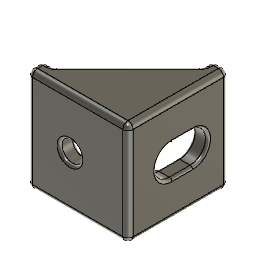
1) Custom PLA Corner Bracket (Autodesk Fusion 360 design; units mm, degrees)
Autodesk Fusion 360 part; units mm, degrees
ref_plane "WorkPlane1" through (0, 0, 0) normal (0, 0, 1) x (1, 0, 0)
sketch "Sketch1" plane through (0, 0, 0) normal (0, 0, 1) x (1, 0, 0)
  line L0 (0, 0) -> (19.5, 0)
  line L1 (19.5, 0) -> (19.5, 19.5)
  line L2 (19.5, 19.5) -> (0, 19.5)
  line L3 (0, 19.5) -> (0, 0)
  line L4 (0, 3) -> (2, 3)
  line L5 (2, 3) -> (16.5, 17.5)
  line L6 (16.5, 17.5) -> (16.5, 19.5)
  dimension "d2" = 19.5
  dimension "d3" = 19.5
  dimension "d4" = 45
  dimension "d5" = 3
  dimension "d7" = 3
  dimension "d8" = 2
  constraint horizontal L0
  constraint vertical L1
  constraint horizontal L2
  constraint vertical L3
  constraint coincident L0.start L3.end
  constraint coincident L3 L4.start
  constraint perpendicular L3 L4
  constraint coincident L2 L6.end
  constraint perpendicular L2 L6
  measures "d2" distance of L0.start L0.end
  measures "d3" distance of L0.start L2.end
  measures "d4" angle of L0 L5
  measures "d5" distance of L1 L6
  measures "d7" distance of L0 L4
  measures "d8" distance of L2 L5.end
extrude "Extrude1" add sketch "Sketch1" along normal blind 3 contours L0 L1 L2 L3 L4 L5 L6
sketch "Sketch2" plane through (0, 0, 3) normal (0, 0, 1) x (-1, 0, 0)
  line L0 (0, -3) -> (0, 0)
  line L1 (0, 0) -> (-19.5, 0)
  line L2 (-19.5, 0) -> (-19.5, -19.5)
  line L3 (-19.5, -19.5) -> (-16.5, -19.5)
  line L4 (-16.5, -19.5) -> (-16.5, -17.5)
  line L5 (-16.5, -17.5) -> (-2, -3)
  line L6 (-2, -3) -> (0, -3)
  line L7 (-2, -3) -> (-16.5, -3)
  line L8 (-16.5, -3) -> (-16.5, -17.5)
  line L9 (-16.5, -17.5) -> (-2, -17.5)
  line L10 (-2, -17.5) -> (-2, -3)
  constraint horizontal L7
  constraint vertical L8
  constraint horizontal L9
  constraint vertical L10
  constraint coincident L4.end L5.start
  constraint coincident L5.end L6.start
extrude "Extrude2" add sketch "Sketch2" along normal blind 14 contours L0 L1 L2 L3 L4 L6 L7 L8
ref_plane "WorkPlane2" through (9.75, 9.75, 17) normal (0, 0, 1) x (1, 0, 0)
sketch "Sketch3" plane through (0, 0, 17) normal (0, 0, 1) x (1, 0, 0)
  line L0 (0, 0) -> (0, 3)
  line L1 (0, 3) -> (2, 3)
  line L2 (2, 3) -> (16.5, 17.5)
  line L3 (16.5, 17.5) -> (16.5, 19.5)
  line L4 (16.5, 19.5) -> (19.5, 19.5)
  line L5 (19.5, 19.5) -> (19.5, 0)
  line L6 (19.5, 0) -> (0, 0)
extrude "Extrude3" add sketch "Sketch3" along normal blind 3
sketch "Sketch4" plane through (16.5, 0, 0) normal (-1, 0, 0) x (0, -1, 0)
  line L0 (-19.5, 0) -> (-17.5, 0)
  line L1 (-17.5, 0) -> (-17.5, 3)
  line L2 (-17.5, 3) -> (-3, 3)
  line L3 (-3, 3) -> (-3, 17)
  line L4 (-3, 17) -> (-17.5, 17)
  line L5 (-17.5, 17) -> (-17.5, 20)
  line L6 (-17.5, 20) -> (-19.5, 20)
  line L7 (-19.5, 20) -> (-19.5, 0)
  line L8 (-15.5, 13) -> (-5.5, 13)
  line L9 (-5.5, 13) -> (-5.5, 7)
  line L10 (-5.5, 7) -> (-15.5, 7)
  line L11 (-15.5, 7) -> (-15.5, 13)
  arc A0 (-8.5, 7) -> (-8.5, 13) centre (-8.5, 10) ccw
  arc A1 (-12.5, 13) -> (-12.5, 7) centre (-12.5, 10) ccw
  line L12 (-10.5, 13) -> (-10.5, 10)
  dimension "d16" = 6
  dimension "d17" = 6
  dimension "d18" = 10
  dimension "d19" = 6
  dimension "d20" = 4
  dimension "d21" = 7
  dimension "d36" = 3
  constraint horizontal L8
  constraint vertical L9
  constraint horizontal L10
  constraint vertical L11
  constraint tangent L8 A1
  constraint tangent L11 A1
  constraint tangent L9 A0
  constraint tangent L8 A0
  constraint coincident L8 A0.end
  constraint coincident L8 A1.start
  constraint coincident L10 A0.start
  constraint coincident L10 A1.end
  constraint midpoint L8 L12.start
  constraint perpendicular L8 L12
  measures "d17" diameter of A0
  measures "d18" distance of L8.start L8.end
  measures "d19" distance of L8.start L10.end
  measures "d20" distance of L7 L11
  measures "d21" distance of L6 L8
  measures "d36" distance of L12.start L12.end
sketch "Sketch5" plane through (0, 3, 0) normal (0, 1, 0) x (-1, 0, 0)
  line L0 (-2, 0) -> (0, 0)
  line L1 (0, 0) -> (0, 20)
  line L2 (0, 20) -> (-2, 20)
  line L3 (-2, 20) -> (-2, 17)
  line L4 (-2, 17) -> (-16.5, 17)
  line L5 (-16.5, 17) -> (-16.5, 3)
  line L6 (-16.5, 3) -> (-2, 3)
  line L7 (-2, 3) -> (-2, 0)
  line L8 (-2, 0) -> (-16.5, 0)
  line L9 (0, 20) -> (-19.5, 20)
  line L10 (0, 0) -> (0, 20)
  line L11 (-16.5, 17) -> (-2, 17)
  line L12 (-2, 17) -> (0, 17)
  line L13 (0, 10) -> (-8.25, 10)
  line L14 (-8.25, 10) -> (-8.25, 17)
  circle A0 centre (-8.25, 10) radius 2
  dimension "d41" = 8.25
  dimension "d42" = 4
  constraint coincident L3.end L4.start
  constraint coincident L1 L12.end
  constraint perpendicular L1 L12
  constraint midpoint L1 L13.start
  constraint perpendicular L1 L13
  constraint coincident L11 L14.end
  constraint perpendicular L11 L14
  constraint coincident L13.end L14.start
  measures "d41" distance of L10 L14
  measures "d42" diameter of A0
extrude "Extrude4" cut sketch "Sketch4" against normal blind 3 contours L8 L10 A0 A1
extrude "Extrude5" cut sketch "Sketch5" against normal blind 3 contours L13 L14 A0 | L13 L14 A0
fillet "Fillet1" radius 1 30 edges at (19.5, 9.75, 0) (9.75, 0, 0) (19.5, 0, 10) (19.5, 9.75, 20) (9.75, 0, 20) (0, 0, 10) (0, 3, 10) (0, 1.5, 20) (0, 1.5, 0) (1, 3, 0) (9.25, 10.25, 0) (16.5, 18.5, 0) (18, 19.5, 0) (16.5, 19.5, 10) (18, 19.5, 20) (16.5, 18.5, 20) (9.25, 10.25, 20) (1, 3, 20) (2, 3, 18.5) (16.5, 17.5, 18.5) (16.5, 17.5, 1.5) (2, 3, 1.5) (16.5, 10.25, 3) (16.5, 3, 10) (16.5, 10.25, 17) (9.25, 3, 17) (9.25, 10.25, 17) (9.25, 10.25, 3) (9.25, 3, 3) (19.5, 19.5, 10)
fillet "Fillet2" radius 0.5 10 edges at (16.5, 10.5, 7) (16.5, 15.5, 10) (16.5, 10.5, 13) (16.5, 5.5, 10) (19.5, 10.5, 13) (19.5, 15.5, 10) (19.5, 10.5, 7) (19.5, 5.5, 10) (10.1147, 0, 9.2768) (10.1147, 3, 10.7232)
ref_plane "WorkPlane3" through (9.75, 9.75, 10) normal (0, 0, 1) x (1, 0, 0)
ref_plane "WorkPlane4" through (9.75, 14, 10) normal (0, -1, 0) x (1, 0, 0)
ref_plane "WorkPlane5" through (5.5, 9.75, 10) normal (1, 0, 0) x (0, 1, 0)
named bodies: "Custom 8020 Corner Bracket"
